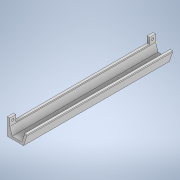
# Autodesk Inventor part: StraightTrackv2
Saved by Autodesk Inventor 2020 (Build 240168000, 168)
## iProperties
Created: 2020-02-27
Part Number: StraightTrackv2
Material: Generic
Document SubType Name: Modeling
Designer: brand
Density: 1 g/cm^3
Appearance: Default
Mass: 15.2552 g
Surface Area: 117.501 cm^2
Volume: 15.2552 cm^3
Author: brand
Autodesk Inventor part; units mm, degrees
ref_plane "YZ Plane" through (0, 0, 0) normal (1, 0, 0) x (0, 1, 0)
ref_plane "XZ Plane" through (0, 0, 0) normal (0, 1, 0) x (-1, 0, 0)
ref_plane "XY Plane" through (0, 0, 0) normal (0, 0, 1) x (1, 0, 0)
sketch "Sketch1" plane through (0, 0, 0) normal (0, 0, 1) x (1, 0, 0)
  circle A0 centre (0, 0) radius 7.62
  line L0 (-7.62, 0) -> (-7.62, 1.27)
  line L1 (0, -7.62) -> (-5.08, -7.62)
  line L2 (0, -7.62) -> (5.08, -7.62)
  line L3 (-7.62, 0) -> (-5.08, -7.62)
  line L4 (5.08, -7.62) -> (7.62, 0)
  line L5 (7.62, 0) -> (7.62, 1.27)
  line L6 (-7.62, 1.27) -> (-10.16, 1.27)
  line L7 (-10.16, 1.27) -> (-10.16, 0)
  line L8 (-5.08, -7.62) -> (-6.7733, -10.16)
  line L9 (-6.7733, -10.16) -> (-10.16, 0)
  line L10 (7.62, 1.27) -> (10.16, 1.27)
  line L11 (10.16, 1.27) -> (10.16, 0)
  line L12 (10.16, 0) -> (6.7733, -10.16)
  line L13 (6.7733, -10.16) -> (-6.7733, -10.16)
  line L14 (5.08, -7.62) -> (6.7733, -10.16)
  dimension "d0" = 15.24
  dimension "d1" = 1.27
  dimension "d2" = 5.08
  dimension "d3" = 5.08
  dimension "d4" = 1.27
  dimension "d6" = 2.54
  dimension "d7" = 2.54
  dimension "d8" = 2.54
  constraints: 30 end point, 4 tangent, 3 equal length, 3 horizontal, 3 point on circle, 3 vertical, 2 parallel, 2 perpendicular, 1 centre point, 1 coincident
  measures "d0" diameter of A0
  measures "d1" distance of L0.start L0.end
  measures "d2" distance of L1.start L1.end
  measures "d3" distance of L1.start L2.end
  measures "d4" distance of L4.end L5.end
  measures "d6" distance of L0.end L6.end
  measures "d7" distance of L5.end L10.end
  measures "d8" distance between parallel lines of L13 L2
extrude "Extrusion1" add sketch "Sketch1" along normal blind 152.4 contours L5 L10 L11 L12 L14 L4 A0 | A0 L4 | L3 A0 | A0 L3 L8 L9 L7 L6 L0 | L2 L14 L13 L8 L1
sketch "Sketch2" plane through (-7.62, 1.27, 152.4) normal (1, 0, 0) x (0, 0, -1)
  point P0 (152.4, -1.27)
sketch "Sketch3" plane through (0, 0, 152.4) normal (0, 0, 1) x (1, 0, 0)
  line L0 (-10.16, 1.27) -> (-10.16, 0) projected
  line L1 (-10.16, 0) -> (-10.16, -10.16)
  line L2 (-6.7733, -10.16) -> (6.7733, -10.16) projected
  line L3 (-10.16, -10.16) -> (-6.7733, -10.16)
  line L4 (-10.16, 0) -> (-6.7733, -10.16) projected
  point P0 (0, 0)
  constraints: 4 end point, 1 horizontal, 1 vertical
extrude "Extrusion2" add sketch "Sketch3" against normal up to surface (152.4 mm away)
sketch "Sketch4" plane through (-7.62, 1.27, 152.4) normal (1, 0, 0) x (0, 0, -1)
  line L0 (152.4, -1.27) -> (152.4, 0) projected
  line L1 (152.4, 0) -> (146.05, 0)
  line L2 (146.05, 0) -> (146.05, 6.35)
  line L3 (146.05, 6.35) -> (152.4, 6.35)
  line L4 (152.4, 6.35) -> (152.4, 0)
  circle A0 centre (149.225, 3.175) radius 1.27
  line L5 (152.4, 0) -> (0, 0) projected
  line L6 (76.2, 0) -> (76.2, 6.35)
  line L7 (76.2, 0) -> (82.55, 0) construction
  line L8 (6.35, 0) -> (6.35, 6.35)
  line L9 (6.35, 6.35) -> (0, 6.35)
  line L10 (0, 6.35) -> (0, 0)
  circle A1 centre (3.175, 3.175) radius 1.27
  dimension "d13" = 6.35
  dimension "d14" = 6.35
  dimension "d15" = 2.54
  dimension "d16" = 3.175
  dimension "d17" = 3.175
  dimension "d18" = 6.35
  dimension "d19" = 90
  constraints: 18 end point, 4 symmetric about line, 2 centre point, 2 horizontal, 2 parallel, 2 perpendicular, 1 midpoint, 1 vertical, 1 other
  measures "d13" distance of L2.end L3.end
  measures "d14" distance of L1.end L2.end
  measures "d15" diameter of A0
  measures "d16" distance from line of L3 A0.centre
  measures "d17" distance from line of L4 A0.centre
  measures "d18" distance of L6.start L6.end
  measures "d19" angle of L7 L6
extrude "Extrusion3" add sketch "Sketch4" against normal up to surface (2.54 mm away)
body "Solid1"
